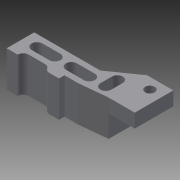
# Autodesk Inventor part: servo_clip_header
Saved by Autodesk Inventor 2015 (Build 190159000, 159)
## iProperties
Created: 2017-12-04
Part Number: servo_clip_header
Material: Generic
Document SubType Name: Modeling
Designer: Anshul
Density: 1 g/cm^3
Appearance: Default
Author: Anshul
Autodesk Inventor part; units mm, degrees
ref_plane "YZ Plane" through (0, 0, 0) normal (1, 0, 0) x (0, 1, 0)
ref_plane "XZ Plane" through (0, 0, 0) normal (0, 1, 0) x (-1, 0, 0)
ref_plane "XY Plane" through (0, 0, 0) normal (0, 0, 1) x (1, 0, 0)
sketch "Sketch1" plane through (0, 0, 0) normal (0, 1, 0) x (-1, 0, 0)
  line L0 (15, 0) -> (15, 8)
  line L1 (15, 8) -> (20, 8)
  line L2 (20, 8) -> (20, 10)
  line L3 (20, 10) -> (25, 10)
  line L4 (25, 10) -> (25, 8)
  line L5 (25, 8) -> (35, 8)
  line L6 (35, 8) -> (35, 10)
  line L7 (35, 10) -> (39, 10)
  line L8 (39, 10) -> (39, 0)
  line L9 (39, 0) -> (15, 0)
  line L10 (15, 4) -> (39, 4)
  line L11 (39, 4) -> (34, 4)
  arc A0 (34, 2) -> (34, 6) centre (34, 4) ccw
  arc A1 (15, 6) -> (15, 2) centre (15, 4) ccw
  line L12 (34, 4) -> (15, 4)
  line L13 (24.5, 4) -> (27.5, 4)
  line L14 (24.5, 4) -> (21.5, 4)
  arc A2 (27.5, 6) -> (27.5, 2) centre (27.5, 4) ccw
  arc A3 (21.5, 2) -> (21.5, 6) centre (21.5, 4) ccw
  line L15 (15, 2) -> (21.5, 2)
  line L16 (27.5, 2) -> (34, 2)
  line L17 (15, 6) -> (21.5, 6)
  line L18 (27.5, 6) -> (34, 6)
  line L19 (5, 7) -> (15, 8)
  line L20 (5, 7) -> (-4.5, 7)
  line L21 (-4.5, 7) -> (-4.5, -3)
  line L22 (-4.5, -3) -> (0, -3)
  circle A4 centre (0, -3) radius 1.75
  line L23 (-4.5, -3) -> (-4.5, -7)
  line L24 (-4.5, -7) -> (5, -7)
  line L25 (5, -7) -> (5, 7)
  line L26 (5, -7) -> (15, 0)
  line L27 (5, 7) -> (9, 7)
  line L28 (9, 7) -> (9, 4)
  line L29 (9, -4.2) -> (9, -0.2)
  arc A5 (11, 4) -> (7, 4) centre (9, 4) ccw
  arc A6 (7, -0.2) -> (11, -0.2) centre (9, -0.2) ccw
  line L30 (7, 4) -> (7, -0.2)
  line L31 (11, -0.2) -> (11, 4)
  line L32 (9, 7) -> (9, 6)
  line L33 (9, -2.2) -> (9, -4.2)
  dimension "d6" = 8
  dimension "d7" = 5
  dimension "d8" = 2
  dimension "d9" = 5
  dimension "d10" = 2
  dimension "d11" = 10
  dimension "d12" = 2
  dimension "d13" = 4
  dimension "d15" = 5
  dimension "d16" = 4
  dimension "d17" = 4
  dimension "d18" = 3
  dimension "d19" = 3
  dimension "d20" = 4
  dimension "d21" = 4
  dimension "d36" = 10
  dimension "d37" = 4.5
  dimension "d38" = 3.5
  dimension "d39" = 4
  dimension "d40" = 4
  dimension "d41" = 3
  dimension "d42" = 4
  dimension "d43" = 4
  dimension "d44" = 4
  constraints: 68 end point, 14 point on circle, 10 perpendicular, 10 point on line, 7 centre point, 7 coincident, 7 tangent, 2 horizontal, 2 midpoint, 2 vertical, 1 collinear
  measures "d6" distance of L0.start L0.end
  measures "d7" distance of L0.end L1.end
  measures "d8" distance of L1.end L2.end
  measures "d9" distance of L2.end L3.end
  measures "d10" distance of L3.end L4.end
  measures "d11" distance of L4.end L5.end
  measures "d12" distance of L5.end L6.end
  measures "d13" distance of L6.end L7.end
  measures "d15" distance of L10.end L11.end
  measures "d16" diameter of A0
  measures "d17" diameter of A1
  measures "d18" distance of L13.start L13.end
  measures "d19" distance of L13.start L14.end
  measures "d20" diameter of A2
  measures "d21" diameter of A3
  measures "d36" distance of L20.end L21.end
  measures "d37" distance of L21.end L22.end
  measures "d38" diameter of A4
  measures "d39" distance of L21.end L23.end
  measures "d40" distance of L19.start L27.end
  measures "d41" distance of L27.end L28.end
  measures "d42" distance of L29.start L29.end
  measures "d43" diameter of A5
  measures "d44" diameter of A6
extrude "Extrusion3" add sketch "Sketch1" against normal blind 8 contours L26 L29 A6 L31 A5 L28 L27 L19 L0 A1 | L0 L15 A3 L10 A2 L16 A0 L8 L9 | L26 L25 L27 L28 A5 L30 A6 L29 | L0 L1 L2 L3 L4 L5 L6 L7 L8 L10 A0 L18 A2 A3 L17
extrude "Extrusion4" add sketch "Sketch1" along normal blind 5 contours L26 L29 A6 L31 A5 L28 L27 L19 L0 A1 | L0 L15 A3 L10 A2 L16 A0 L8 L9 | L26 L25 L27 L28 A5 L30 A6 L29 | L0 L1 L2 L3 L4 L5 L6 L7 L8 L10 A0 L18 A2 A3 L17 | L24 L23 L21 L20 L25
fillet "Fillet2" radius 2 3 edges at (-25, -1.5, 8) (-25, -1.5, 10) (-35, -1.5, 8)
body "Solid2"
